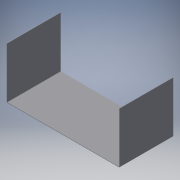
# Autodesk Inventor part: Cup Holder Sheet Metal
Saved by Autodesk Inventor 2019 (Build 230136000, 136)
## iProperties
Created: 2020-12-25
Part Number: Cup Holder Sheet Metal
Material: Generic
Document SubType Name: Sheet Metal
Designer: John
Density: 1 g/cm^3
Sheet Metal Rule: Default
Appearance: Default
Author: John
Autodesk Inventor part; units mm, degrees
ref_plane "YZ Plane" through (0, 0, 0) normal (1, 0, 0) x (0, 1, 0)
ref_plane "XZ Plane" through (0, 0, 0) normal (0, 1, 0) x (-1, 0, 0)
ref_plane "XY Plane" through (0, 0, 0) normal (0, 0, 1) x (1, 0, 0)
sketch "Sketch1" plane through (0, 0, 0) normal (0, 1, 0) x (-1, 0, 0)
  line L0 (-304.8, 76.2) -> (304.8, 76.2)
  line L1 (304.8, 76.2) -> (304.8, -76.2)
  line L2 (304.8, -76.2) -> (-304.8, -76.2)
  line L3 (-304.8, -76.2) -> (-304.8, 76.2)
  line L4 (-304.8, 76.2) -> (304.8, -76.2) construction
  line L5 (304.8, 76.2) -> (-304.8, -76.2) construction
  point P0 (0, 0)
  dimension "d0" = 609.6
  dimension "d1" = 152.4
  measures "d0" distance of L1.end L2.end
  measures "d1" distance of L0.end L1.end
extrude "Plate1" add sketch "Sketch1" along normal blind 1.016
sketch "Sketch2" plane through (0, 0, 0) normal (0, -1, 0) x (1, 0, 0)
  line L0 (304.8, -76.2) -> (304.8, 76.2) projected
  line L1 (304.8, 0) -> (159.7343, 0) construction
  line L2 (159.7343, -76.2) -> (159.7342, 76.2)
  line L3 (-304.8, -76.2) -> (304.8, -76.2) projected
  point P0 (0, 0)
  dimension "d3" = 145.0658
  dimension "d4" = 90
  constraints: 4 end point, 2 midpoint, 1 horizontal, 1 point on line
  measures "d3" distance of L1.end L1.start
  measures "d4" angle of L3 L2
fold "Fold1" angle 90 bend radius 1.016 thickness 1.016 k factor 0.44 line from (159.7343, 0, -76.2) to (159.7342, 0, 76.2) line at bend centre moving side (-1, 0, 0) folds toward (0, 1, 0)
sketch "Sketch5" plane through (159.8673, 2.032, -76.2) normal (1, 0, 0) x (0, 0, -1)
  line L0 (-165.1, 317.373) -> (-165.1, 317.9445)
  line L1 (-152.4, 0) -> (0, 0) projected
  line L2 (0, 463.3852) -> (0, 0) projected
  line L3 (-152.4, 463.3852) -> (0, 463.3852) projected
  line L4 (-152.4, 0) -> (-152.4, 463.3852) projected
  line L5 (0, 463.3852) -> (0, 0) projected
  line L6 (0, 318.3194) -> (-152.4, 318.3194)
  line L7 (-152.4, 0) -> (-152.4, 463.3852) projected
  point P0 (-76.2, -2.032)
  dimension "d31" = 145.0658
  constraints: 4 end point, 2 point on line, 1 perpendicular, 1 vertical, 2 other
  measures "d31" distance between parallel lines of L3 L6
fold "Fold4" angle 90 bend radius 1.016 thickness 1.016 k factor 0.44 line from (159.8673, 320.3514, -76.2) to (159.8673, 320.3514, 76.2) line at bend centre moving side (0, -1, 0) folds toward (1, 0, 0)
sketch "Sketch6" plane through (160.8833, 319.4685, -76.2) normal (0, -1, 0) x (1, 0, 0)
  line L0 (0, 152.4) -> (0, 0) projected
  line L1 (0, 0) -> (317.1704, 0) projected
  line L2 (317.1704, 0) -> (317.1704, 152.4) projected
  line L3 (317.1704, 152.4) -> (0, 152.4) projected
  line L4 (0, 0) -> (317.1704, 0) projected
  line L5 (158.5852, 0) -> (158.5852, 152.4)
  line L6 (234.7852, 76.2) -> (82.3852, 76.2) construction
  circle A0 centre (82.3852, 76.2) radius 57.15
  circle A1 centre (234.7852, 76.2) radius 57.15
  point P0 (-160.8833, 76.2)
  point P1 (158.5852, 76.2)
  dimension "d32" = 152.4
  dimension "d33" = 114.3
  constraints: 4 end point, 4 midpoint, 2 centre point, 2 coincident, 1 equal radius, 1 horizontal
  measures "d32" distance of L6.start L6.end
  measures "d33" diameter of A0
extrude "Cut1" cut sketch "Sketch6" against normal blind 1.016 contours A0 | A1
equation "\"d2\" = Thickness"
equation "\"d5\" = BendReliefWidth"
equation "\"d6\" = BendReliefDepth"
equation "\"d7\" = MinimumRemnant"
equation "\"d8\" = TransitionRadius"
equation "\"d10\" = BendRadius"
equation "\"d25\" = BendReliefWidth"
equation "\"d26\" = BendReliefDepth"
equation "\"d27\" = MinimumRemnant"
equation "\"d28\" = TransitionRadius"
equation "\"d30\" = BendRadius"
equation "\"d35\" = Thickness"
equation "\"BendRadius\" = Thickness"
equation "\"BendReliefWidth\" = Thickness"
equation "\"BendReliefDepth\" = 0.5 * Thickness"
equation "\"CornerReliefSize\" = 4 * Thickness"
equation "\"MinimumRemnant\" = 2 * Thickness"
equation "\"TransitionRadius\" = BendRadius"
equation "\"JacobiRadiusSize\" = BendRadius"
equation "\"GapSize\" = Thickness"
equation "\"Thickness\" = 1.016"
body "Solid1"
